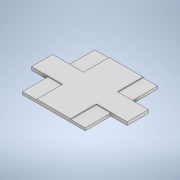
# Autodesk Inventor part: Podkladka
Saved by Autodesk Inventor 2022 (Build 260153000, 153)
## iProperties
Created: 2023-08-16
Part Number: Podkladka
Material: Generic
Document SubType Name: Modeling
Designer: Kippi
Density: 1 g/cm^3
Appearance: Default
Author: Kippi
Autodesk Inventor part; units mm, degrees
ref_plane "YZ Plane" through (0, 0, 0) normal (1, 0, 0) x (0, 1, 0)
ref_plane "XZ Plane" through (0, 0, 0) normal (0, 1, 0) x (-1, 0, 0)
ref_plane "XY Plane" through (0, 0, 0) normal (0, 0, 1) x (1, 0, 0)
sketch "Sketch1" plane through (0, 0, 0) normal (0, 1, 0) x (-1, 0, 0)
  line L0 (86.4286, 125.7143) -> (-104.5714, 125.7143)
  line L1 (-104.5714, 125.7143) -> (-104.5714, -94.2857)
  line L2 (-104.5714, -94.2857) -> (86.4286, -94.2857)
  line L3 (86.4286, -94.2857) -> (86.4286, 125.7143)
  point P0 (0, 0)
  dimension "d0" = 220
  dimension "d1" = 191
  constraints: 8 end point, 2 parallel, 1 horizontal, 1 perpendicular
  measures "d0" distance of L2.end L0.start
  measures "d1" distance of L1.end L2.end
extrude "Extrusion1" add sketch "Sketch1" along normal blind 10
sketch "Sketch2" plane through (0, 10, 0) normal (0, 1, 0) x (1, 0, 0)
  line L0 (104.5714, -125.7143) -> (104.5714, 94.2857) construction
  line L1 (104.5714, 94.2857) -> (-86.4286, 94.2857) construction
  line L2 (-86.4286, 94.2857) -> (-86.4286, -125.7143) construction
  line L3 (-86.4286, -125.7143) -> (104.5714, -125.7143) construction
  line L4 (-86.4286, -125.7143) -> (-42.4286, -125.7143)
  line L5 (-42.4286, -125.7143) -> (-42.4286, -47.7143)
  line L6 (-42.4286, -47.7143) -> (-86.4286, -47.7143)
  line L7 (-86.4286, -47.7143) -> (-86.4286, -125.7143)
  line L8 (-86.4286, 94.2857) -> (-42.4286, 94.2857)
  line L9 (-42.4286, 94.2857) -> (-42.4286, 16.2857)
  line L10 (-42.4286, 16.2857) -> (-86.4286, 16.2857)
  line L11 (-86.4286, 16.2857) -> (-86.4286, 94.2857)
  line L12 (104.5714, 94.2857) -> (60.5714, 94.2857)
  line L13 (60.5714, 94.2857) -> (60.5714, 16.2857)
  line L14 (60.5714, 16.2857) -> (104.5714, 16.2857)
  line L15 (104.5714, 16.2857) -> (104.5714, 94.2857)
  line L16 (104.5714, -125.7143) -> (60.5714, -125.7143)
  line L17 (60.5714, -125.7143) -> (60.5714, -47.7143)
  line L18 (60.5714, -47.7143) -> (104.5714, -47.7143)
  line L19 (104.5714, -47.7143) -> (104.5714, -125.7143)
  point P0 (0, 0)
  dimension "d4" = 191
  dimension "d5" = 220
  dimension "d6" = 78
  dimension "d7" = 78
  dimension "d8" = 78
  dimension "d9" = 78
  dimension "d10" = 44
  dimension "d11" = 44
  dimension "d12" = 44
  dimension "d13" = 44
  constraints: 32 end point, 8 parallel, 4 horizontal, 4 perpendicular, 1 point on line
  measures "d4" distance of point (-86.429, -125.714) point (104.571, -125.714)
  measures "d5" distance of point (-86.429, 94.286) point (-86.429, -125.714)
  measures "d6" distance of L4.end L5.end
  measures "d7" distance of L16.end L17.end
  measures "d8" distance of L12.end L13.end
  measures "d9" distance of L8.end L9.end
  measures "d10" distance of L5.end L6.end
  measures "d11" distance of L9.end L10.end
  measures "d12" distance of L13.end L14.end
  measures "d13" distance of L17.end L18.end
extrude "Extrusion2" cut sketch "Sketch2" against normal blind 2
sketch "Sketch4" plane through (0, 10, 0) normal (0, 1, 0) x (1, 0, 0)
  line L0 (-86.4286, 16.2857) -> (-86.4286, -47.7143) construction
  line L1 (104.5714, -47.7143) -> (104.5714, 16.2857) construction
  line L2 (-136.4286, -47.7143) -> (154.5714, -47.7143)
  line L3 (154.5714, -47.7143) -> (154.5714, 16.2857)
  line L4 (154.5714, 16.2857) -> (-136.4286, 16.2857)
  line L5 (-136.4286, 16.2857) -> (-136.4286, -47.7143)
  point P0 (0, 0)
  dimension "d18" = 50
  dimension "d19" = 50
  constraints: 8 end point, 2 parallel, 1 horizontal, 1 perpendicular
  measures "d18" distance between parallel lines of L5 L0
  measures "d19" distance between parallel lines of L1 L3
extrude "Extrusion4" add sketch "Sketch4" against normal blind 10
body "Solid1"
